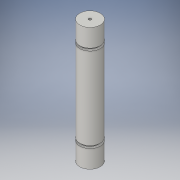
# Autodesk Inventor part: Roller
Saved by Autodesk Inventor 2016 (Build 200138000, 138)
## iProperties
Created: 2016-01-18
Part Number: Roller
Material: PVC-Piping
Document SubType Name: Modeling
Designer: yash
Density: 1.4 g/cm^3
Appearance: Smooth - White
Author: yash
Autodesk Inventor part; units mm, degrees
ref_plane "YZ Plane" through (0, 0, 0) normal (1, 0, 0) x (0, 1, 0)
ref_plane "XZ Plane" through (0, 0, 0) normal (0, 1, 0) x (-1, 0, 0)
ref_plane "XY Plane" through (0, 0, 0) normal (0, 0, 1) x (1, 0, 0)
sketch "Sketch1" plane through (0, 0, 0) normal (0, 0, 1) x (1, 0, 0)
  line L0 (0, 0) -> (25.4, 0)
  line L1 (25.4, 304.8) -> (0, 304.8)
  line L2 (0, 304.8) -> (0, 0)
  line L3 (25.4, 44.45) -> (19.05, 44.45)
  line L4 (19.05, 44.45) -> (19.05, 50.8)
  line L5 (19.05, 50.8) -> (25.4, 50.8)
  line L6 (25.4, 254) -> (19.05, 254)
  line L7 (19.05, 254) -> (19.05, 260.35)
  line L8 (19.05, 260.35) -> (25.4, 260.35)
  line L9 (25.4, 260.35) -> (25.4, 304.8)
  line L10 (25.4, 0) -> (25.4, 44.45)
  line L11 (25.4, 50.8) -> (25.4, 254)
  point P0 (12.7, 152.4)
  point P1 (12.7, 0)
  dimension "d3" = 6.35
  dimension "d4" = 6.35
  dimension "d5" = 6.35
  dimension "d7" = 6.35
  dimension "d8" = 25.4
  dimension "d9" = 25.4
  dimension "d10" = 25.4
  dimension "d11" = 304.8
  dimension "d12" = 152.4
  dimension "d13" = 101.6
  dimension "d14" = 101.6
  constraints: 24 end point, 6 parallel, 5 perpendicular, 3 horizontal, 1 midpoint, 1 vertical alignment
  measures "d3" distance between parallel lines of L11 L7
  measures "d4" distance of L6.end L7.end
  measures "d5" distance between parallel lines of L5 L3
  measures "d7" distance between parallel lines of L10 L4
  measures "d8" distance between parallel lines of L2 L10
  measures "d9" distance between parallel lines of L2 L11
  measures "d10" distance between parallel lines of L2 L9
  measures "d11" distance of L1.end L0.start
  measures "d12" distance from line of L1 point (12.7, 152.4)
  measures "d13" distance from line of L6 point (12.7, 152.4)
  measures "d14" distance from line of L5 point (12.7, 152.4)
revolve "Revolution1" add sketch "Sketch1" angle 360 about axis through (0, 304.8, 0) along (0, -1, 0)
sketch "Sketch2" plane through (0, 304.8, 0) normal (0, 1, 0) x (1, 0, 0)
  point P0 (0, 0)
  point P1 (0, 0)
  constraints: 1 coincident
hole "Hole1" at (0, 304.8, 0) direction (0, -1, 0) diameter 6.604 end through all
equation "\"d12\" = 0.5 * d11"
body "Solid1"
